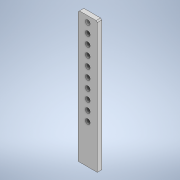
# Autodesk Inventor part: graduated_foot_03
Saved by Autodesk Inventor 2020 (Build 240168000, 168)
## iProperties
Created: 2019-12-19
Part Number: graduated_foot_03
Material: Générique
Document SubType Name: Modeling
Designer: damien
Density: 1 g/cm^3
Appearance: Par défaut
Author: damien
Autodesk Inventor part; units mm, degrees
ref_plane "YZ Plane" through (0, 0, 0) normal (1, 0, 0) x (0, 1, 0)
ref_plane "XZ Plane" through (0, 0, 0) normal (0, 1, 0) x (-1, 0, 0)
ref_plane "XY Plane" through (0, 0, 0) normal (0, 0, 1) x (1, 0, 0)
sketch "Esquisse1" plane through (0, 0, 0) normal (0, 0, 1) x (1, 0, 0)
  line L0 (0, 0) -> (80, 0)
  line L1 (80, 0) -> (80, 550)
  line L2 (80, 550) -> (0, 550)
  line L3 (0, 550) -> (0, 0)
  dimension "d0" = 80
  dimension "d1" = 550
  constraints: 8 end point, 2 parallel, 1 horizontal, 1 perpendicular
  measures "d0" distance of L0.start L0.end
  measures "d1" distance of L2.end L0.start
extrude "Extrusion1" add sketch "Esquisse1" along normal blind 18.55
sketch "Esquisse2" plane through (0, 0, 18.55) normal (0, 0, 1) x (1, 0, 0)
  line L0 (80, 550) -> (0, 550) projected
  line L1 (40, 550) -> (40, 0) construction
  circle A0 centre (40, 525) radius 10
  circle A1 centre (40, 485) radius 10
  circle A2 centre (40, 445) radius 10
  circle A3 centre (40, 405) radius 10
  circle A4 centre (40, 365) radius 10
  circle A5 centre (40, 325) radius 10
  circle A6 centre (40, 285) radius 10
  circle A7 centre (40, 245) radius 10
  circle A8 centre (40, 205) radius 10
  circle A9 centre (40, 165) radius 10
  point P0 (0, 0)
  dimension "d4" = 25
  dimension "d5" = 20
  dimension "d8" = 40
  constraints: 10 centre point, 2 end point, 2 vertical, 1 midpoint, 1 point on line, 18 other
  measures "d4" distance from line of A0.centre L0
  measures "d5" diameter of A0
  measures "d8" distance of A0.centre A1.centre
extrude "Extrusion2" cut sketch "Esquisse2" against normal blind 18.55
chamfer "Chanfrein1" distance 5 angle 45 2 edges at (0, 550, 9.275) (80, 550, 9.275)
